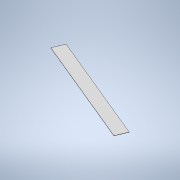
# Autodesk Inventor part: balsa sheet
Saved by Autodesk Inventor 2022 (Build 260153000, 153)
## iProperties
Created: 2021-06-25
Part Number: balsa sheet
Material: Generic
Document SubType Name: Modeling
Designer: Ferdinand Hubbard
Density: 1 g/cm^3
Appearance: Default
Author: Ferdinand Hubbard
Autodesk Inventor part; units mm, degrees
ref_plane "YZ Plane" through (0, 0, 0) normal (1, 0, 0) x (0, 1, 0)
ref_plane "XZ Plane" through (0, 0, 0) normal (0, 1, 0) x (-1, 0, 0)
ref_plane "XY Plane" through (0, 0, 0) normal (0, 0, 1) x (1, 0, 0)
sketch "Sketch1" plane through (0, 0, 0) normal (0, 1, 0) x (-1, 0, 0)
  line L0 (0, 0) -> (923.8795, -382.6834)
  line L1 (923.8795, -382.6834) -> (962.1479, -290.2955)
  line L2 (962.1479, -290.2955) -> (38.2683, 92.388)
  line L3 (38.2683, 92.388) -> (0, 0)
  line L4 (0, 0) -> (1000, 0) construction
  dimension "d2" = 1000
  dimension "d3" = 22.5
  dimension "d4" = 100
  constraints: 10 end point, 2 parallel, 1 equal length, 1 horizontal, 1 perpendicular
  measures "d2" distance of L0.start L0.end
  measures "d3" angle of L0 L4
  measures "d4" distance of L1.end L0.end
extrude "Extrusion1" add sketch "Sketch1" along normal blind 2
body "Solid1"
